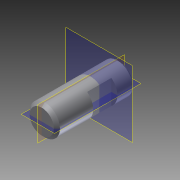
# Autodesk Inventor part: TU-011
Saved by Autodesk Inventor 2011 (Build 150229000, 229)
## iProperties
Shininess: 64.0
Angle Display Precision: 2
Document Length Units: 11269
Document Angle Units: 11279
Document Time Units: 11290
Document Mass Units: 11283
Document Length Units Precision: 3
Document Angle Units Precision: 2
Compacted: True
Created: 2002-07-24
Part Number: TU-011
Document SubType Name: Modeling
Designer: PN
Description: Lock Pin
Density: 1 g/cm^3
Mass: 1.92325 g
Surface Area: 9.46666 cm^2
Volume: 1.92325 cm^3
Density: 0.0
Volumn: 0.0
Area: 0.0
PropertySet Name: Model Information
Control State: 0
Master: False
Checked Out: False
Author: PN
Autodesk Inventor part; units mm, degrees
ref_plane "XY Plane" through (0, 0, 0) normal (0, 0, 1) x (1, 0, 0)
sketch "Sketch1" plane through (0, 0, 0) normal (0, 0, 1) x (1, 0, 0)
  circle A0 centre (0, 0) radius 5
  dimension "d0" = 10
  constraints: 1 centre point, 1 coincident
  measures "d0" diameter of A0
extrude "Extrusion1" add sketch "Sketch1" along normal mid plane 26
chamfer "Chamfer1" distance 1 angle 45 2 edges at (-5, 0, 13) (-5, 0, -13)
sketch "Sketch2" plane through (0, 0, 0) normal (0, 1, 0) x (-1, 0, 0)
  line L0 (-5, -12) -> (-5, 12) projected
  line L1 (-5, 7) -> (-3, 7)
  line L2 (-3, 7) -> (-3, -1)
  line L3 (-3, -1) -> (-5, -1)
  line L4 (-5, -1) -> (-5, 7)
  line L5 (-4, 13) -> (4, 13) projected
  dimension "d5" = 2
  dimension "d6" = 8
  dimension "d7" = 6
  constraints: 8 end point, 2 parallel, 1 horizontal, 1 perpendicular, 1 point on line
  measures "d5" distance of L1.start L1.end
  measures "d6" distance of L1.end L2.end
  measures "d7" distance between parallel lines of L1 L5
extrude "Extrusion2" cut sketch "Sketch2" along normal through all both and the other way through all
ref_plane "Work Plane1" through (3, -4, 3) normal (0, 0, 1) x (1, 0, 0)
body "Solid1"
